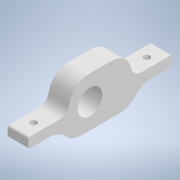
# Autodesk Inventor part: BearingBlocks
Saved by Autodesk Inventor 2021 (Build 250183000, 183)
## iProperties
Created: 2021-05-22
Part Number: BearingBlocks
Material: Generic
Document SubType Name: Modeling
Designer: sami8
Density: 1 g/cm^3
Appearance: Default
Author: sami8
Autodesk Inventor part; units mm, degrees
ref_plane "YZ Plane" through (0, 0, 0) normal (1, 0, 0) x (0, 1, 0)
ref_plane "XZ Plane" through (0, 0, 0) normal (0, 1, 0) x (-1, 0, 0)
ref_plane "XY Plane" through (0, 0, 0) normal (0, 0, 1) x (1, 0, 0)
sketch "Sketch1" plane through (0, 0, 0) normal (1, 0, 0) x (0, 1, 0)
  line L0 (0, 0) -> (-5, 0)
  line L1 (-5, 0) -> (-5, -20)
  line L2 (-5, -20) -> (0, -20)
  line L3 (0, -20) -> (0, 0)
  line L4 (-12, -20) -> (12, -20)
  line L5 (12, -20) -> (12, -50)
  line L6 (12, -50) -> (-12, -50)
  line L7 (-12, -50) -> (-12, -20)
  circle A0 centre (0.5, -34) radius 6
  line L8 (0.5, -19.8614) -> (0.5, -49.8614) construction
  line L9 (0, -50) -> (-5, -50)
  line L10 (-5, -50) -> (-5, -70)
  line L11 (-5, -70) -> (0, -70)
  line L12 (0, -70) -> (0, -50)
  point P0 (0, -20)
  dimension "d0" = 5
  dimension "d1" = 20
  dimension "d7" = 24
  dimension "d8" = 30
  dimension "d9" = 12
  dimension "d10" = 7
  dimension "d11" = 14
  dimension "d12" = 5
  dimension "d13" = 20
  dimension "d26" = 12.5
  constraints: 26 end point, 6 parallel, 3 horizontal, 3 perpendicular, 1 centre point, 1 collinear, 1 midpoint, 1 point on line
  measures "d0" distance of L2.end L1.end
  measures "d1" distance of L1.end L0.end
  measures "d7" distance of L5.end L6.end
  measures "d8" distance of L6.end L4.start
  measures "d9" diameter of A0
  measures "d10" distance between parallel lines of L1 L7
  measures "d11" distance from line of L4 A0.centre
  measures "d12" distance of L11.end L10.end
  measures "d13" distance of L10.end L9.end
  measures "d26" distance between parallel lines of L8 L7
extrude "Extrusion1" add sketch "Sketch1" along normal blind 8.7
sketch "Sketch2" plane through (0, -5, 0) normal (0, -1, 0) x (1, 0, 0)
  line L0 (0, 0) -> (8.7, 0) projected
  line L1 (4.35, 0) -> (4.35, -7.5) construction
  circle A0 centre (4.35, -7.5) radius 1.55
  line L2 (0, -70) -> (8.7, -70) projected
  line L3 (4.35, -70) -> (4.35, -62.5) construction
  circle A1 centre (4.35, -62.5) radius 1.55
  dimension "d17" = 7.5
  dimension "d18" = 3.1
  dimension "d19" = 7.5
  dimension "d20" = 3.1
  constraints: 4 end point, 2 centre point, 2 coincident, 2 midpoint, 2 vertical
  measures "d17" distance of L1.start L1.end
  measures "d18" diameter of A0
  measures "d19" distance of L3.start L3.end
  measures "d20" diameter of A1
extrude "Extrusion2" cut sketch "Sketch2" against normal through all
fillet "Fillet2" radius 10 6 edges at (4.35, 12, -20) (4.35, 12, -50) (4.35, -12, -50) (4.35, -5, -50) (4.35, -5, -20) (4.35, -12, -20)
fillet "Fillet2" radius 5 2 edges at (4.35, 0, -20) (4.35, 0, -50)
fillet "Fillet2" radius 1 4 edges at (4.35, 0, -70) (4.35, -5, -70) (4.35, 0, 0) (4.35, -5, 0)
body "Solid1"
